Autodesk Inventor part; units mm, degrees
(part 2 of 2)
  spline S15 degree 3 poles (2.6737, 15.108) (2.737, 15.0887) (2.7959, 15.0572) (2.8984, 14.9734) (2.941, 14.922) (3.0039, 14.8056) (3.0237, 14.7419) (3.0386, 14.6027) (3.0287, 14.545) (2.9716, 14.2674) (2.9092, 14.0596) (2.9838, 13.6157) (3.0427, 13.4596) (3.2171, 13.1787) (3.3308, 13.0566) (3.6259, 12.8434) (3.773, 12.7944) (4.1825, 12.6632) (4.4508, 12.5425) (4.8985, 12.5133) (5.0632, 12.5344) (5.3764, 12.6389) (5.5216, 12.7214) (5.7403, 12.91) (5.8538, 13.0253) (6.0406, 13.397) (6.0705, 13.5567) (6.2474, 13.7265) (6.3037, 13.7625) (6.4211, 13.8087) (6.4805, 13.8206) (6.6006, 13.8232) (6.6604, 13.8138) (6.7172, 13.7941) knots 0 0 0 0 0.019863 0.019863 0.03972 0.03972 0.059573 0.059573 0.081705 0.081705 0.153115 0.153115 0.194508 0.194508 0.235922 0.235922 0.285548 0.285548 0.382717 0.382717 0.438735 0.438735 0.494976 0.494976 0.536961 0.536961 0.576712 0.576712 0.591396 0.591396 0.604738 0.604738 0.618079 0.618079 0.618079 0.618079
  line L495 (2.6737, 15.108) -> (2.737, 15.0887) construction
  line L496 (2.737, 15.0887) -> (2.7959, 15.0572) construction
  line L497 (2.7959, 15.0572) -> (2.8984, 14.9734) construction
  line L498 (2.8984, 14.9734) -> (2.941, 14.922) construction
  line L499 (2.941, 14.922) -> (3.0039, 14.8056) construction
  line L500 (3.0039, 14.8056) -> (3.0237, 14.7419) construction
  line L501 (3.0237, 14.7419) -> (3.0386, 14.6027) construction
  line L502 (3.0386, 14.6027) -> (3.0287, 14.545) construction
  line L503 (3.0287, 14.545) -> (2.9716, 14.2674) construction
  line L504 (2.9716, 14.2674) -> (2.9092, 14.0596) construction
  line L505 (2.9092, 14.0596) -> (2.9838, 13.6157) construction
  line L506 (2.9838, 13.6157) -> (3.0427, 13.4596) construction
  line L507 (3.0427, 13.4596) -> (3.2171, 13.1787) construction
  line L508 (3.2171, 13.1787) -> (3.3308, 13.0566) construction
  line L509 (3.3308, 13.0566) -> (3.6259, 12.8434) construction
  line L510 (3.6259, 12.8434) -> (3.773, 12.7944) construction
  line L511 (3.773, 12.7944) -> (4.1825, 12.6632) construction
  line L512 (4.1825, 12.6632) -> (4.4508, 12.5425) construction
  line L513 (4.4508, 12.5425) -> (4.8985, 12.5133) construction
  line L514 (4.8985, 12.5133) -> (5.0632, 12.5344) construction
  line L515 (5.0632, 12.5344) -> (5.3764, 12.6389) construction
  line L516 (5.3764, 12.6389) -> (5.5216, 12.7214) construction
  line L517 (5.5216, 12.7214) -> (5.7403, 12.91) construction
  line L518 (5.7403, 12.91) -> (5.8538, 13.0253) construction
  line L519 (5.8538, 13.0253) -> (6.0406, 13.397) construction
  line L520 (6.0406, 13.397) -> (6.0705, 13.5567) construction
  line L521 (6.0705, 13.5567) -> (6.2474, 13.7265) construction
  line L522 (6.2474, 13.7265) -> (6.3037, 13.7625) construction
  line L523 (6.3037, 13.7625) -> (6.4211, 13.8087) construction
  line L524 (6.4211, 13.8087) -> (6.4805, 13.8206) construction
  line L525 (6.4805, 13.8206) -> (6.6006, 13.8232) construction
  line L526 (6.6006, 13.8232) -> (6.6604, 13.8138) construction
  line L527 (6.6604, 13.8138) -> (6.7172, 13.7941) construction
  arc A16 (7.2114, 13.5423) -> (6.7172, 13.7941) centre (0, 0) ccw
  spline S16 degree 3 poles (7.2114, 13.5423) (7.2657, 13.5044) (7.312, 13.4563) (7.3836, 13.3449) (7.4082, 13.2828) (7.4321, 13.1527) (7.4312, 13.0859) (7.4024, 12.949) (7.3751, 12.8972) (7.235, 12.6509) (7.1115, 12.4725) (7.0452, 12.0272) (7.053, 11.8606) (7.1321, 11.5395) (7.2025, 11.3883) (7.4173, 11.0944) (7.542, 11.0023) (7.8909, 10.751) (8.1088, 10.5533) (8.5256, 10.3871) (8.6887, 10.3563) (9.0189, 10.3589) (9.1825, 10.3925) (9.4488, 10.5043) (9.5924, 10.5789) (9.8848, 10.8746) (9.9626, 11.0174) (10.1834, 11.1241) (10.248, 11.1409) (10.374, 11.1486) (10.4341, 11.1416) (10.5491, 11.1069) (10.6031, 11.0795) (10.6511, 11.0433) knots 0 0 0 0 0.019863 0.019863 0.03972 0.03972 0.059573 0.059573 0.081705 0.081705 0.153115 0.153115 0.194508 0.194508 0.235922 0.235922 0.285548 0.285548 0.382717 0.382717 0.438735 0.438735 0.494976 0.494976 0.536961 0.536961 0.576712 0.576712 0.591396 0.591396 0.604738 0.604738 0.618079 0.618079 0.618079 0.618079
  line L528 (7.2114, 13.5423) -> (7.2657, 13.5044) construction
  line L529 (7.2657, 13.5044) -> (7.312, 13.4563) construction
  line L530 (7.312, 13.4563) -> (7.3836, 13.3449) construction
  line L531 (7.3836, 13.3449) -> (7.4082, 13.2828) construction
  line L532 (7.4082, 13.2828) -> (7.4321, 13.1527) construction
  line L533 (7.4321, 13.1527) -> (7.4312, 13.0859) construction
  line L534 (7.4312, 13.0859) -> (7.4024, 12.949) construction
  line L535 (7.4024, 12.949) -> (7.3751, 12.8972) construction
  line L536 (7.3751, 12.8972) -> (7.235, 12.6509) construction
  line L537 (7.235, 12.6509) -> (7.1115, 12.4725) construction
  line L538 (7.1115, 12.4725) -> (7.0452, 12.0272) construction
  line L539 (7.0452, 12.0272) -> (7.053, 11.8606) construction
  line L540 (7.053, 11.8606) -> (7.1321, 11.5395) construction
  line L541 (7.1321, 11.5395) -> (7.2025, 11.3883) construction
  line L542 (7.2025, 11.3883) -> (7.4173, 11.0944) construction
  line L543 (7.4173, 11.0944) -> (7.542, 11.0023) construction
  line L544 (7.542, 11.0023) -> (7.8909, 10.751) construction
  line L545 (7.8909, 10.751) -> (8.1088, 10.5533) construction
  line L546 (8.1088, 10.5533) -> (8.5256, 10.3871) construction
  line L547 (8.5256, 10.3871) -> (8.6887, 10.3563) construction
  line L548 (8.6887, 10.3563) -> (9.0189, 10.3589) construction
  line L549 (9.0189, 10.3589) -> (9.1825, 10.3925) construction
  line L550 (9.1825, 10.3925) -> (9.4488, 10.5043) construction
  line L551 (9.4488, 10.5043) -> (9.5924, 10.5789) construction
  line L552 (9.5924, 10.5789) -> (9.8848, 10.8746) construction
  line L553 (9.8848, 10.8746) -> (9.9626, 11.0174) construction
  line L554 (9.9626, 11.0174) -> (10.1834, 11.1241) construction
  line L555 (10.1834, 11.1241) -> (10.248, 11.1409) construction
  line L556 (10.248, 11.1409) -> (10.374, 11.1486) construction
  line L557 (10.374, 11.1486) -> (10.4341, 11.1416) construction
  line L558 (10.4341, 11.1416) -> (10.5491, 11.1069) construction
  line L559 (10.5491, 11.1069) -> (10.6031, 11.0795) construction
  line L560 (10.6031, 11.0795) -> (10.6511, 11.0433) construction
  arc A17 (11.0433, 10.6511) -> (10.6511, 11.0433) centre (0, 0) ccw
  spline S17 degree 3 poles (11.0433, 10.6511) (11.0832, 10.5982) (11.1124, 10.5381) (11.146, 10.4101) (11.1502, 10.3435) (11.1327, 10.2123) (11.1113, 10.1491) (11.0415, 10.0277) (10.9996, 9.987) (10.7903, 9.7959) (10.6176, 9.6645) (10.417, 9.2615) (10.373, 9.1006) (10.3489, 8.7708) (10.3692, 8.6052) (10.4826, 8.2593) (10.5728, 8.1332) (10.8269, 7.7864) (10.9731, 7.531) (11.3181, 7.2442) (11.4638, 7.1645) (11.7786, 7.0649) (11.9445, 7.0464) (12.2323, 7.0704) (12.3919, 7.0969) (12.7615, 7.2878) (12.8796, 7.3995) (13.1225, 7.4328) (13.1891, 7.4289) (13.3113, 7.3972) (13.3664, 7.372) (13.465, 7.3034) (13.5079, 7.2607) (13.5423, 7.2114) knots 0 0 0 0 0.019863 0.019863 0.03972 0.03972 0.059573 0.059573 0.081705 0.081705 0.153115 0.153115 0.194508 0.194508 0.235922 0.235922 0.285548 0.285548 0.382717 0.382717 0.438735 0.438735 0.494976 0.494976 0.536961 0.536961 0.576712 0.576712 0.591396 0.591396 0.604738 0.604738 0.618079 0.618079 0.618079 0.618079
  line L561 (11.0433, 10.6511) -> (11.0832, 10.5982) construction
  line L562 (11.0832, 10.5982) -> (11.1124, 10.5381) construction
  line L563 (11.1124, 10.5381) -> (11.146, 10.4101) construction
  line L564 (11.146, 10.4101) -> (11.1502, 10.3435) construction
  line L565 (11.1502, 10.3435) -> (11.1327, 10.2123) construction
  line L566 (11.1327, 10.2123) -> (11.1113, 10.1491) construction
  line L567 (11.1113, 10.1491) -> (11.0415, 10.0277) construction
  line L568 (11.0415, 10.0277) -> (10.9996, 9.987) construction
  line L569 (10.9996, 9.987) -> (10.7903, 9.7959) construction
  line L570 (10.7903, 9.7959) -> (10.6176, 9.6645) construction
  line L571 (10.6176, 9.6645) -> (10.417, 9.2615) construction
  line L572 (10.417, 9.2615) -> (10.373, 9.1006) construction
  line L573 (10.373, 9.1006) -> (10.3489, 8.7708) construction
  line L574 (10.3489, 8.7708) -> (10.3692, 8.6052) construction
  line L575 (10.3692, 8.6052) -> (10.4826, 8.2593) construction
  line L576 (10.4826, 8.2593) -> (10.5728, 8.1332) construction
  line L577 (10.5728, 8.1332) -> (10.8269, 7.7864) construction
  line L578 (10.8269, 7.7864) -> (10.9731, 7.531) construction
  line L579 (10.9731, 7.531) -> (11.3181, 7.2442) construction
  line L580 (11.3181, 7.2442) -> (11.4638, 7.1645) construction
  line L581 (11.4638, 7.1645) -> (11.7786, 7.0649) construction
  line L582 (11.7786, 7.0649) -> (11.9445, 7.0464) construction
  line L583 (11.9445, 7.0464) -> (12.2323, 7.0704) construction
  line L584 (12.2323, 7.0704) -> (12.3919, 7.0969) construction
  line L585 (12.3919, 7.0969) -> (12.7615, 7.2878) construction
  line L586 (12.7615, 7.2878) -> (12.8796, 7.3995) construction
  line L587 (12.8796, 7.3995) -> (13.1225, 7.4328) construction
  line L588 (13.1225, 7.4328) -> (13.1891, 7.4289) construction
  line L589 (13.1891, 7.4289) -> (13.3113, 7.3972) construction
  line L590 (13.3113, 7.3972) -> (13.3664, 7.372) construction
  line L591 (13.3664, 7.372) -> (13.465, 7.3034) construction
  line L592 (13.465, 7.3034) -> (13.5079, 7.2607) construction
  line L593 (13.5079, 7.2607) -> (13.5423, 7.2114) construction
  arc A18 (13.7941, 6.7172) -> (13.5423, 7.2114) centre (0, 0) ccw
  spline S18 degree 3 poles (13.7941, 6.7172) (13.8158, 6.6546) (13.8249, 6.5884) (13.8174, 6.4563) (13.8008, 6.3916) (13.7436, 6.2723) (13.7037, 6.2188) (13.5999, 6.1249) (13.5474, 6.0991) (13.2893, 5.9821) (13.0845, 5.9105) (12.7691, 5.5892) (12.6775, 5.4498) (12.5527, 5.1435) (12.5209, 4.9798) (12.5218, 4.6158) (12.5686, 4.468) (12.7031, 4.0596) (12.7632, 3.7715) (13.0028, 3.3921) (13.1166, 3.2713) (13.3853, 3.0794) (13.5374, 3.0104) (13.8185, 2.9443) (13.9785, 2.9203) (14.3889, 2.9876) (14.5358, 3.0573) (14.7771, 3.0139) (14.8393, 2.9896) (14.9457, 2.9218) (14.9902, 2.8807) (15.0629, 2.7851) (15.0904, 2.7312) (15.108, 2.6737) knots 0 0 0 0 0.019863 0.019863 0.03972 0.03972 0.059573 0.059573 0.081705 0.081705 0.153115 0.153115 0.194508 0.194508 0.235922 0.235922 0.285548 0.285548 0.382717 0.382717 0.438735 0.438735 0.494976 0.494976 0.536961 0.536961 0.576712 0.576712 0.591396 0.591396 0.604738 0.604738 0.618079 0.618079 0.618079 0.618079
  line L594 (13.7941, 6.7172) -> (13.8158, 6.6546) construction
  line L595 (13.8158, 6.6546) -> (13.8249, 6.5884) construction
  line L596 (13.8249, 6.5884) -> (13.8174, 6.4563) construction
  line L597 (13.8174, 6.4563) -> (13.8008, 6.3916) construction
  line L598 (13.8008, 6.3916) -> (13.7436, 6.2723) construction
  line L599 (13.7436, 6.2723) -> (13.7037, 6.2188) construction
  line L600 (13.7037, 6.2188) -> (13.5999, 6.1249) construction
  line L601 (13.5999, 6.1249) -> (13.5474, 6.0991) construction
  line L602 (13.5474, 6.0991) -> (13.2893, 5.9821) construction
  line L603 (13.2893, 5.9821) -> (13.0845, 5.9105) construction
  line L604 (13.0845, 5.9105) -> (12.7691, 5.5892) construction
  line L605 (12.7691, 5.5892) -> (12.6775, 5.4498) construction
  line L606 (12.6775, 5.4498) -> (12.5527, 5.1435) construction
  line L607 (12.5527, 5.1435) -> (12.5209, 4.9798) construction
  line L608 (12.5209, 4.9798) -> (12.5218, 4.6158) construction
  line L609 (12.5218, 4.6158) -> (12.5686, 4.468) construction
  line L610 (12.5686, 4.468) -> (12.7031, 4.0596) construction
  line L611 (12.7031, 4.0596) -> (12.7632, 3.7715) construction
  line L612 (12.7632, 3.7715) -> (13.0028, 3.3921) construction
  line L613 (13.0028, 3.3921) -> (13.1166, 3.2713) construction
  line L614 (13.1166, 3.2713) -> (13.3853, 3.0794) construction
  line L615 (13.3853, 3.0794) -> (13.5374, 3.0104) construction
  line L616 (13.5374, 3.0104) -> (13.8185, 2.9443) construction
  line L617 (13.8185, 2.9443) -> (13.9785, 2.9203) construction
  line L618 (13.9785, 2.9203) -> (14.3889, 2.9876) construction
  line L619 (14.3889, 2.9876) -> (14.5358, 3.0573) construction
  line L620 (14.5358, 3.0573) -> (14.7771, 3.0139) construction
  line L621 (14.7771, 3.0139) -> (14.8393, 2.9896) construction
  line L622 (14.8393, 2.9896) -> (14.9457, 2.9218) construction
  line L623 (14.9457, 2.9218) -> (14.9902, 2.8807) construction
  line L624 (14.9902, 2.8807) -> (15.0629, 2.7851) construction
  line L625 (15.0629, 2.7851) -> (15.0904, 2.7312) construction
  line L626 (15.0904, 2.7312) -> (15.108, 2.6737) construction
  arc A19 (15.1947, 2.1258) -> (15.108, 2.6737) centre (0, 0) ccw
  spline S19 degree 3 poles (15.1947, 2.1258) (15.196, 2.0596) (15.1842, 1.9938) (15.1362, 1.8705) (15.1004, 1.8141) (15.0092, 1.7183) (14.9547, 1.6797) (14.827, 1.6226) (14.7691, 1.6142) (14.4874, 1.5827) (14.2705, 1.5779) (13.8713, 1.3697) (13.7411, 1.2655) (13.5278, 1.0128) (13.4469, 0.8669) (13.3353, 0.5204) (13.3341, 0.3654) (13.3359, -0.0646) (13.304, -0.3571) (13.4146, -0.792) (13.4856, -0.942) (13.6817, -1.2076) (13.8051, -1.3202) (14.052, -1.4699) (14.1967, -1.5423) (14.6079, -1.605) (14.7691, -1.5841) (14.9852, -1.7) (15.0368, -1.7423) (15.1171, -1.8397) (15.1468, -1.8925) (15.1863, -2.0059) (15.1958, -2.0657) (15.1947, -2.1258) knots 0 0 0 0 0.019863 0.019863 0.03972 0.03972 0.059573 0.059573 0.081705 0.081705 0.153115 0.153115 0.194508 0.194508 0.235922 0.235922 0.285548 0.285548 0.382717 0.382717 0.438735 0.438735 0.494976 0.494976 0.536961 0.536961 0.576712 0.576712 0.591396 0.591396 0.604738 0.604738 0.618079 0.618079 0.618079 0.618079
  line L627 (15.1947, 2.1258) -> (15.196, 2.0596) construction
  line L628 (15.196, 2.0596) -> (15.1842, 1.9938) construction
  line L629 (15.1842, 1.9938) -> (15.1362, 1.8705) construction
  line L630 (15.1362, 1.8705) -> (15.1004, 1.8141) construction
  line L631 (15.1004, 1.8141) -> (15.0092, 1.7183) construction
  line L632 (15.0092, 1.7183) -> (14.9547, 1.6797) construction
  line L633 (14.9547, 1.6797) -> (14.827, 1.6226) construction
  line L634 (14.827, 1.6226) -> (14.7691, 1.6142) construction
  line L635 (14.7691, 1.6142) -> (14.4874, 1.5827) construction
  line L636 (14.4874, 1.5827) -> (14.2705, 1.5779) construction
  line L637 (14.2705, 1.5779) -> (13.8713, 1.3697) construction
  line L638 (13.8713, 1.3697) -> (13.7411, 1.2655) construction
  line L639 (13.7411, 1.2655) -> (13.5278, 1.0128) construction
  line L640 (13.5278, 1.0128) -> (13.4469, 0.8669) construction
  line L641 (13.4469, 0.8669) -> (13.3353, 0.5204) construction
  line L642 (13.3353, 0.5204) -> (13.3341, 0.3654) construction
  line L643 (13.3341, 0.3654) -> (13.3359, -0.0646) construction
  line L644 (13.3359, -0.0646) -> (13.304, -0.3571) construction
  line L645 (13.304, -0.3571) -> (13.4146, -0.792) construction
  line L646 (13.4146, -0.792) -> (13.4856, -0.942) construction
  line L647 (13.4856, -0.942) -> (13.6817, -1.2076) construction
  line L648 (13.6817, -1.2076) -> (13.8051, -1.3202) construction
  line L649 (13.8051, -1.3202) -> (14.052, -1.4699) construction
  line L650 (14.052, -1.4699) -> (14.1967, -1.5423) construction
  line L651 (14.1967, -1.5423) -> (14.6079, -1.605) construction
  line L652 (14.6079, -1.605) -> (14.7691, -1.5841) construction
  line L653 (14.7691, -1.5841) -> (14.9852, -1.7) construction
  line L654 (14.9852, -1.7) -> (15.0368, -1.7423) construction
  line L655 (15.0368, -1.7423) -> (15.1171, -1.8397) construction
  line L656 (15.1171, -1.8397) -> (15.1468, -1.8925) construction
  line L657 (15.1468, -1.8925) -> (15.1863, -2.0059) construction
  line L658 (15.1863, -2.0059) -> (15.1958, -2.0657) construction
  line L659 (15.1958, -2.0657) -> (15.1947, -2.1258) construction
  point P0 (13.5417, -7.2124)
  point P1 (13.7941, -6.7172)
  point P2 (15.1076, -2.6748)
  point P3 (15.1948, -2.1189)
  point P4 (15.1948, 2.1247)
  point P5 (15.108, 2.6737)
  point P6 (13.7945, 6.7161)
  point P7 (11.044, 10.6501)
  point P8 (10.6511, 11.0433)
  point P9 (7.2124, 13.5417)
  point P10 (6.7172, 13.7941)
  point P11 (2.6748, 15.1076)
  point P12 (-2.1247, 15.1948)
  point P13 (-2.6737, 15.108)
  point P14 (-6.7161, 13.7945)
  point P15 (-10.6501, 11.044)
  point P16 (-11.0433, 10.6511)
  point P17 (-13.5417, 7.2124)
  point P18 (-13.7941, 6.7172)
  point P19 (-15.1076, 2.6748)
  point P20 (-15.1948, -2.1247)
  point P21 (-15.108, -2.6737)
  point P22 (-13.7945, -6.7161)
  point P23 (-13.5383, -7.217)
  point P24 (-11.044, -10.6501)
  point P25 (-10.6511, -11.0433)
  point P26 (-7.2124, -13.5417)
  point P27 (-6.7172, -13.7941)
  point P28 (-2.6748, -15.1076)
  point P29 (2.1247, -15.1948)
  point P30 (2.6737, -15.108)
  point P31 (6.7161, -13.7945)
  point P32 (10.6501, -11.044)
  point P33 (11.0433, -10.6511)
  constraints: 40 point on circle, 20 centre point, 1480 other
extrude "Extrusion1" add sketch "Sketch1" along normal mid plane 10
sketch "Sketch2" plane through (0, -5, 0) normal (0, -1, 0) x (1, 0, 0)
  circle A0 centre (0, 0) radius 16.8275
  dimension "d2" = 33.655
  constraints: 1 centre point, 1 coincident
  measures "d2" diameter of A0
extrude "Extrusion2" add sketch "Sketch2" along normal blind 1.5875
chamfer "Chamfer1" distance 0.7937 angle 45 1 edges at (-16.8275, -5, 0)
mirror "Mirror1" about plane through (0, 0, 0) normal (0, 1, 0) of "Extrusion2", "Chamfer1"
sketch "Sketch7" plane through (0, 6.5875, 0) normal (0, 1, 0) x (1, 0, 0)
  point P0 (0, 0)
hole "Hole2" at (0, 6.5875, 0) direction (0, -1, 0) diameter 19.05 end through all
sketch "Sketch3" plane through (0, -6.5875, 0) normal (0, -1, 0) x (1, 0, 0)
  circle A0 centre (0, 0) radius 7.9375
  dimension "d8" = 15.875
  constraints: 1 centre point, 1 coincident
  measures "d8" diameter of A0
sketch "Sketch4" plane through (0, 6.5875, 0) normal (0, 1, 0) x (1, 0, 0)
  circle A0 centre (0, 0) radius 4.7625
  dimension "d11" = 9.525
  constraints: 1 centre point, 1 coincident
  measures "d11" diameter of A0
sketch "Sketch5" plane through (0, 7.6035, 0) normal (0, 1, 0) x (1, 0, 0)
  point P0 (0, 0)
  point P1 (0, 0)
  constraints: 1 coincident
body "Solid1"
